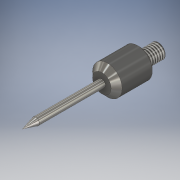
# Autodesk Inventor part: carbide_probe_30deg_tip_r02
Saved by Autodesk Inventor 2016 SP1 (Build 200210100, 210)
## iProperties
Created: 2016-06-29
Part Number: carbide_probe_30deg_tip_r02
Material: Steel, High Strength, Low Alloy
Document SubType Name: Modeling
Designer: Stephen Holtz
Density: 7.85 g/cm^3
Appearance: Steel - Polished
Vendor: Carbide Probes
Author: Stephen Holtz
Title: Carbide Antenna Probe 30 Degree Taper
Autodesk Inventor part; units mm, degrees
ref_plane "YZ Plane" through (0, 0, 0) normal (1, 0, 0) x (0, 1, 0)
ref_plane "XZ Plane" through (0, 0, 0) normal (0, 1, 0) x (-1, 0, 0)
ref_plane "XY Plane" through (0, 0, 0) normal (0, 0, 1) x (1, 0, 0)
sketch "Sketch1" plane through (0, 0, 0) normal (0, 1, 0) x (-1, 0, 0)
  line L0 (0, 0) -> (-3.05, 0)
  line L1 (-3.05, 0) -> (-3.05, -7.62)
  line L2 (-3.05, -7.62) -> (0, -7.62)
  line L3 (0, -7.62) -> (0, 0)
  line L4 (0, 0) -> (-0.762, 0)
  line L5 (-0.762, 0) -> (-0.762, 13.6652)
  line L6 (-0.762, 13.6652) -> (0, 13.6652)
  line L7 (0, 13.6652) -> (0, 0)
  line L8 (-0.762, 13.6652) -> (0, 16.509)
  line L9 (-0.762, 13.6652) -> (2.1821, 13.6652) construction
  line L10 (0, 16.509) -> (0, 13.6652)
  dimension "d0" = 3.05
  dimension "d1" = 7.62
  dimension "d2" = 0.762
  dimension "d3" = 13.6652
  dimension "d13" = 75
  dimension "d14" = 15
  dimension "d15" = 16.509
  dimension "d16" = 24.129
  constraints: 22 end point, 4 parallel, 3 horizontal, 3 perpendicular, 1 equal length
  measures "d0" distance of L2.end L1.end
  measures "d1" distance of L1.end L0.end
  measures "d2" distance of L5.end L6.end
  measures "d3" distance of L4.end L5.end
  measures "d13" angle of L9 L8
  measures "d14" angle of L10 L8
  measures "d15" distance of L0.start L8.end
  measures "d16" distance of L2.end L8.end
revolve "Revolution1" add sketch "Sketch1" angle 360 about axis through (0, 0, 13.6652) along (0, 0, -1)
sketch "Sketch2" plane through (0, 0, -7.62) normal (0, 0, -1) x (-1, 0, 0)
  circle A0 centre (0, 0) radius 3.05 projected
  circle A1 centre (0, 0) radius 1.5
  dimension "d5" = 3
  constraints: 1 centre point, 1 coincident
  measures "d5" diameter of A1
extrude "Extrusion1" add sketch "Sketch2" along normal blind 4 contours A1
chamfer "Chamfer1" distance 1.143 angle 45 1 edges at (-3.05, 0, 0)
chamfer "Chamfer2" distance 0.254 angle 45 1 edges at (-3.05, 0, -7.62)
thread "Thread1" size "M3x0.5" class "6g" standard "ANSI Metric M Profile" full length
body "Solid1"
